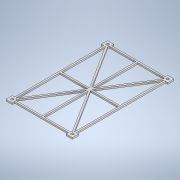
# Autodesk Inventor part: WedgeDrillGuideV3.2
Saved by Autodesk Inventor 2020 (Build 240168000, 168)
## iProperties
Created: 2023-12-20
Part Number: WedgeDrillGuideV3.2
Material: Generic
Document SubType Name: Modeling
Designer: smz3rm
Density: 1 g/cm^3
Appearance: Default
Author: smz3rm
Autodesk Inventor part; units mm, degrees
ref_plane "YZ Plane" through (0, 0, 0) normal (1, 0, 0) x (0, 1, 0)
ref_plane "XZ Plane" through (0, 0, 0) normal (0, 1, 0) x (-1, 0, 0)
ref_plane "XY Plane" through (0, 0, 0) normal (0, 0, 1) x (1, 0, 0)
sketch "Sketch1" plane through (0, 0, 0) normal (0, 1, 0) x (-1, 0, 0)
  line L0 (-42.5, 65) -> (42.5, 65)
  line L1 (42.5, 65) -> (42.5, -65)
  line L2 (42.5, -65) -> (-42.5, -65)
  line L3 (-42.5, -65) -> (-42.5, 65)
  line L4 (-42.5, 65) -> (42.5, -65) construction
  line L5 (42.5, 65) -> (-42.5, -65) construction
  line L6 (42.5, 65) -> (34.5, 65)
  line L7 (34.5, 65) -> (34.5, 57)
  line L8 (34.5, 57) -> (42.5, 57)
  line L9 (42.5, 57) -> (42.5, 65)
  line L10 (42.5, -65) -> (34.5, -65)
  line L11 (34.5, -65) -> (34.5, -57)
  line L12 (34.5, -57) -> (42.5, -57)
  line L13 (42.5, -57) -> (42.5, -65)
  line L14 (-42.5, 65) -> (-34.5, 65)
  line L15 (-34.5, 65) -> (-34.5, 57)
  line L16 (-34.5, 57) -> (-42.5, 57)
  line L17 (-42.5, 57) -> (-42.5, 65)
  line L18 (-42.5, -65) -> (-34.5, -65)
  line L19 (-34.5, -65) -> (-34.5, -57)
  line L20 (-34.5, -57) -> (-42.5, -57)
  line L21 (-42.5, -57) -> (-42.5, -65)
  circle A0 centre (38.5, 61) radius 1.6
  line L22 (34.5, 61) -> (42.5, 61)
  line L23 (38.5, 57) -> (38.5, 65)
  line L24 (34.5, -61) -> (42.5, -61)
  line L25 (38.5, -57) -> (38.5, -65)
  line L26 (-34.5, 61) -> (-42.5, 61)
  line L27 (-38.5, 57) -> (-38.5, 65)
  line L28 (-34.5, -61) -> (-42.5, -61)
  line L29 (-38.5, -57) -> (-38.5, -65)
  circle A1 centre (-38.5, -61) radius 1.6
  circle A2 centre (-38.5, 61) radius 1.6
  circle A3 centre (38.5, -61) radius 1.6
  circle A4 centre (38.5, 61) radius 3.6
  circle A5 centre (38.5, -61) radius 3.6
  circle A6 centre (-38.5, 61) radius 3.6
  circle A7 centre (-38.5, -61) radius 3.6
  line L30 (35.0417, 62) -> (-35.0417, 62)
  line L31 (35.0417, 60) -> (-35.0417, 60)
  line L32 (59.5, 0) -> (-59.5, 0) projected
  line L33 (0, -91) -> (0, 91) projected
  line L34 (35.0417, -62) -> (-35.0417, -62)
  line L35 (35.0417, -60) -> (-35.0417, -60)
  line L36 (39.5, 57.5417) -> (39.5, -57.5417)
  line L37 (37.5, 57.5417) -> (37.5, -57.5417)
  line L38 (-39.5, 57.5417) -> (-39.5, -57.5417)
  line L39 (-37.5, 57.5417) -> (-37.5, -57.5417)
  line L40 (38.5, 61) -> (-38.5, -61)
  line L41 (-38.5, 61) -> (38.5, -61)
  line L42 (-39.3457, 60.4663) -> (37.6543, -61.5337)
  line L43 (-37.6543, 61.5337) -> (39.3457, -60.4663)
  line L44 (39.3457, 60.4663) -> (-37.6543, -61.5337)
  line L45 (37.6543, 61.5337) -> (-39.3457, -60.4663)
  line L46 (1, 60) -> (1, 3.458)
  line L47 (-1, 60) -> (-1, 3.458)
  line L48 (1, -3.458) -> (1, -60)
  line L49 (-1, -3.458) -> (-1, -60)
  line L50 (37.5, 1) -> (1.8137, 1)
  line L51 (37.5, -1) -> (1.8137, -1)
  line L52 (-37.5, 1) -> (-1.8137, 1)
  line L53 (-37.5, -1) -> (-1.8137, -1)
  point P0 (0, 0)
  point P1 (-39.5, 57.5417)
  point P2 (-35.0417, -62)
  point P3 (37.5, 57.5417)
  point P4 (37.5, -57.5417)
  point P5 (-37.5, 57.5417)
  point P6 (-35.0417, 60)
  point P7 (-1.1825, 0)
  point P8 (-37.5, -57.542)
  point P9 (-35.8085, -58.6092)
  point P10 (0, -1.8736)
  point P11 (35.8085, -58.6092)
  point P12 (37.5, -57.542)
  point P13 (1.1825, 0)
  point P14 (37.5, 57.542)
  point P15 (35.8085, 58.6092)
  point P16 (0, 1.8736)
  point P17 (-35.8085, 58.6092)
  point P18 (-37.5, 57.542)
  point P19 (38.5, 64.6)
  point P20 (42.1, 61)
  point P21 (-34.5, 62)
  point P22 (-39.5, 57)
  point P23 (-39.5, -57)
  point P24 (-34.5, -62)
  point P25 (39.5, -57)
  point P26 (34.5, -62)
  point P27 (39.5, 57)
  point P28 (34.5, 62)
  point P29 (-1, 3.458)
  point P30 (-37.4998, -57.5417)
  point P31 (-37.4998, 57.5417)
  point P32 (37.4998, 57.5417)
  point P33 (37.4998, -57.5417)
  dimension "d0" = 85
  dimension "d1" = 130
  dimension "d2" = 8
  dimension "d3" = 3.2
  dimension "d4" = 2
  dimension "d5" = 2
  dimension "d6" = 2
  dimension "d7" = 2
  dimension "d8" = 2
  dimension "d9" = 2
  dimension "d12" = 1
  dimension "d13" = 1
  dimension "d14" = 1
  dimension "d15" = 1
  dimension "d16" = 2
  dimension "d17" = 2
  constraints: 104 end point, 23 midpoint, 20 symmetric about line, 16 parallel, 9 point on line, 7 perpendicular, 6 centre point, 6 equal length, 5 horizontal, 3 equal radius, 2 collinear, 2 point on circle, 2 vertical, 1 coincident, 6 other
  measures "d0" distance of L1.end L2.end
  measures "d1" distance of L0.end L1.end
  measures "d2" distance of L8.end L7.end
  measures "d3" diameter of A0
  measures "d4" radial gap between concentric circles of A0 A4
  measures "d7" radial gap between concentric circles of A1 A7
  measures "d8" distance between parallel lines of L31 L30
  measures "d9" distance between parallel lines of L37 L36
  measures "d12" distance between parallel lines of L41 L42
  measures "d13" distance between parallel lines of L41 L43
  measures "d14" distance between parallel lines of L40 L44
  measures "d15" distance between parallel lines of L40 L45
  measures "d16" distance between parallel lines of L47 L46
  measures "d17" distance between parallel lines of L51 L50
extrude "Extrusion1" add sketch "Sketch1" along normal blind 2 contours L0 L27 A6 L26 L3 | L0 L15 L30 A6 L27 | L26 A6 L38 L16 L3 | A6 L26 A2 L27 | L27 A2 L26 A6 | L26 A2 L42 L27 A6 | L30 L33 L31 L15 | L15 L26 A6 L30 | L38 A6 L27 L16 | L16 L39 L32 L38 | L0 L23 A4 L30 L7 | L30 L7 L31 L33 | L15 L31 A6 L26 | L26 A6 L43 A2 | L20 L38 A7 L28 L3 | L32 L39 L20 L38 | L27 A6 L39 L16 | A2 L27 L42 | L27 L42 A6 | L0 L1 L22 A4 L23 | L30 A4 L22 L7 | L33 L43 L47 L31 | L31 L46 L45 L33 | A2 L41 A6 L42 L27 | A2 L43 A6 L41 | L28 A7 L29 L2 L3 | L20 L29 A7 L38 | L39 L52 L42 L32 | L32 L45 L53 L39 | A6 L41 L16 L42 | A4 L22 A0 L23 | L23 A0 L22 A4 | L22 A4 L31 L7 | L43 L40 L33 | L45 L41 L16 L43 | L45 L8 L40 L43 | L33 L41 L45 | A6 L43 L16 L41 | A7 L29 L45 A1 L28 | L28 A1 L29 A7 | L20 L39 A7 L29 | L45 L41 L32 | L32 L40 L42 | L42 L16 L41 L45 | L42 L40 L20 L45 | L1 L8 L36 A4 L22 | A4 L23 L44 A0 L22 | L22 A0 L45 A4 | L40 L43 L32 | L41 L44 L33 | L33 L42 L40 | L32 L44 L41 | L40 L8 L44 L43 | L29 A7 L34 L19 L2 | L29 A1 L28 A7 | A7 L45 L29 | L42 L44 L20 L40 | L36 L8 L23 A4 | L45 A4 L40 L8 | L44 L50 L37 L32 | L32 L37 L51 L43 | L43 L12 L41 L44 | L42 L48 L35 L33 | L44 L41 L12 L42 | L33 L35 L49 L44 | L40 A4 L44 L8 | L45 L29 A1 | A7 L28 L19 L34 | L20 L40 A7 L45 | A7 L40 A1 L29 L45 | L20 L44 A7 L40 | L36 L32 L37 L8 | L44 L23 A0 | A0 L40 A4 L45 | L23 L44 A4 L40 A0 | A4 L44 L23 | L23 L8 L37 A4 | L32 L36 L12 L37 | L35 L11 L34 L33 | L33 L34 L19 L35 | L41 A5 L42 L12 | L12 L43 A5 L41 | L40 A7 L44 A1 | A1 L44 A7 L28 | A7 L35 L19 L28 | L1 L24 A5 L36 L12 | L41 A3 L42 A5 | A5 L43 L25 A3 L41 | L11 L34 A5 L25 L2 | L1 L2 L25 A5 L24 | L36 A5 L25 L12 | L12 L25 A5 L37 | A5 L25 L43 | L11 L24 A5 L34 | L35 A5 L24 L11 | L42 A3 L24 A5 | A5 L25 A3 L24 | L24 A3 L43 L25 A5 | L43 A3 L25 | A5 L24 A3 L25
equation "\"d0\" = BoxLength"
equation "\"d1\" = BoxWidth"
equation "\"d2\" = M3ScrewInsertBrim"
equation "\"BoxLength\" = 85"
equation "\"BoxWidth\" = 130"
equation "\"M3ScrewInsertBrim\" = 8"
body "Solid1"
